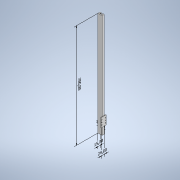
# Autodesk Inventor part: Guia
Saved by Autodesk Inventor 2021 (Build 250183000, 183)
## iProperties
Created: 2021-08-09
Part Number: Guia
Material: Generic
Document SubType Name: Modeling
Designer: guilh
Density: 1 g/cm^3
Appearance: Default
Author: guilh
Autodesk Inventor part; units mm, degrees
ref_plane "YZ Plane" through (0, 0, 0) normal (1, 0, 0) x (0, 1, 0)
ref_plane "XZ Plane" through (0, 0, 0) normal (0, 1, 0) x (-1, 0, 0)
ref_plane "XY Plane" through (0, 0, 0) normal (0, 0, 1) x (1, 0, 0)
sketch "Sketch1" plane through (0, 0, 0) normal (0, 1, 0) x (-1, 0, 0)
  line L0 (0, 0) -> (16, 0)
  line L1 (16, 0) -> (16, -5)
  line L2 (16, -5) -> (12, -5)
  line L3 (12, -5) -> (12, -10)
  line L4 (12, -10) -> (22, -10)
  line L5 (22, -10) -> (22, 5)
  line L6 (22, 5) -> (-4, 5)
  line L7 (0, 0) -> (0, -5)
  line L8 (0, -5) -> (4, -5)
  line L9 (4, -5) -> (4, -10)
  line L10 (4, -10) -> (-6, -10)
  line L11 (-6, -10) -> (-6, 5)
  line L12 (-6, 5) -> (-4, 5)
  dimension "d0" = 16
  dimension "d1" = 5
  dimension "d2" = 4
  dimension "d3" = 5
  dimension "d4" = 10
  dimension "d5" = 15
  dimension "d6" = 26
  dimension "d11" = 5
  dimension "d12" = 4
  dimension "d13" = 5
  dimension "d14" = 10
  dimension "d15" = 15
  constraints: 26 end point, 9 perpendicular, 2 vertical, 1 horizontal
  measures "d0" distance of L0.start L0.end
  measures "d1" distance of L0.end L1.end
  measures "d2" distance of L1.end L2.end
  measures "d3" distance of L2.end L3.end
  measures "d4" distance of L3.end L4.end
  measures "d5" distance of L4.end L5.end
  measures "d6" distance of L5.end L6.end
  measures "d11" distance of L0.start L7.end
  measures "d12" distance of L7.end L8.end
  measures "d13" distance of L8.end L9.end
  measures "d14" distance of L9.end L10.end
  measures "d15" distance of L10.end L11.end
extrude "Extrusion1" add sketch "Sketch1" along normal blind 500
sketch "Sketch2" plane through (6, 0, 5) normal (1, 0, 0) x (0, 0, -1)
  line L0 (0, 0) -> (0, 500) projected
  line L1 (0, 0) -> (0, 80)
  line L2 (0, 80) -> (15, 80)
  line L3 (15, 0) -> (15, 500) projected
  line L4 (15, 80) -> (35, 80)
  line L5 (35, 80) -> (35, 110)
  line L6 (35, 110) -> (-20, 110)
  line L7 (-20, 110) -> (-20, 50)
  line L8 (-20, 50) -> (35, 50)
  line L9 (35, 50) -> (35, 80)
  line L10 (-20, 110) -> (-10, 110)
  line L11 (-10, 110) -> (-10, 90)
  line L12 (-10, 90) -> (-10, 70)
  line L13 (-10, 70) -> (25, 70)
  line L14 (25, 70) -> (25, 90)
  line L15 (-10, 95) -> (-15.9639, 95)
  line L16 (-10, 65) -> (-17.5959, 65)
  circle A0 centre (25, 95) radius 5
  circle A1 centre (-10, 95) radius 5
  circle A2 centre (25, 65) radius 5
  circle A3 centre (-10, 65) radius 5
  point P0 (5, 0)
  dimension "d18" = 80
  dimension "d19" = 15
  dimension "d20" = 20
  dimension "d21" = 30
  dimension "d22" = 55
  dimension "d23" = 60
  dimension "d24" = 10
  dimension "d25" = 20
  dimension "d26" = 20
  dimension "d27" = 35
  dimension "d28" = 20
  dimension "d33" = 10
  dimension "d34" = 10
  dimension "d35" = 10
  dimension "d36" = 10
  constraints: 30 end point, 8 perpendicular, 7 point on line, 4 centre point, 1 horizontal
  measures "d18" distance of L0.start L1.end
  measures "d19" distance of L1.end L2.end
  measures "d20" distance of L2.end L4.end
  measures "d21" distance of L4.end L5.end
  measures "d22" distance of L5.end L6.end
  measures "d23" distance of L6.end L7.end
  measures "d24" distance of L6.end L10.end
  measures "d25" distance of L10.end L11.end
  measures "d26" distance of L11.end L12.end
  measures "d27" distance of L12.end L13.end
  measures "d28" distance of L13.end L14.end
  measures "d33" diameter of A0
  measures "d34" diameter of A1
  measures "d35" diameter of A2
  measures "d36" diameter of A3
extrude "Extrusion2" add sketch "Sketch2" along normal blind 3 contours L8 L7 L6 L11 A1 L12 L13 L0 | L0 L13 L3 L8 | L13 L12 A1 L11 L6 L0 | L0 L2 L3 L13 | L3 L13 L14 L4 L9 L8 | L0 L6 L3 L2 | L3 L4 L14 L13 | L3 L6 L5 L4
sketch "Sketch3" plane through (6, 0, 5) normal (-1, 0, 0) x (0, 0, 1)
  line L0 (20, 50) -> (-35, 50) projected
  line L1 (-35, 50) -> (-35, 110) projected
  line L2 (-35, 50) -> (-35, 110)
  line L3 (-35, 110) -> (20, 110) projected
  line L4 (-35, 110) -> (20, 110)
  line L5 (20, 110) -> (20, 50) projected
  line L6 (20, 110) -> (20, 50)
  line L7 (20, 50) -> (-35, 50)
  point P0 (-5, 0)
  constraints: 8 end point, 2 perpendicular, 1 collinear, 1 vertical
extrude "Extrusion3" add sketch "Sketch3" against normal blind 3
sketch "Sketch4" plane through (6, 0, 5) normal (-1, 0, 0) x (0, 0, 1)
  line L0 (0, 50) -> (0, 110) projected
  line L1 (0, 50) -> (9, 50)
  line L2 (20, 50) -> (-35, 50) projected
  line L3 (9, 50) -> (9, 110)
  line L4 (-35, 110) -> (20, 110) projected
  line L5 (9, 110) -> (23.2747, 110)
  line L6 (-35, 110) -> (-15, 110) projected
  line L7 (23.2747, 110) -> (23.2747, 50)
  line L8 (23.2747, 50) -> (9, 50)
  line L9 (-15, 50) -> (-35, 50) projected
  line L10 (-15, 50) -> (-24, 50)
  line L11 (-24, 50) -> (-24, 110)
  line L12 (-24, 110) -> (-51.0156, 108.7427)
  line L13 (-51.0156, 108.7427) -> (-51.1782, 112.2347)
  line L14 (-51.1782, 112.2347) -> (-24, 110)
  line L15 (-51.0156, 108.7427) -> (-55.6093, 34.9275)
  line L16 (-55.6093, 34.9275) -> (-24, 50)
  point P0 (-5, 0)
  dimension "d41" = 9
  dimension "d42" = 9
  constraints: 24 end point, 5 point on line, 4 perpendicular, 2 collinear
  measures "d41" distance of L0.start L1.end
  measures "d42" distance of L9.start L10.end
extrude "Extrusion4" cut sketch "Sketch4" against normal blind 3 contours L3 L4 L5 L7 L8 L2 | L16 L15 L12 L11 | L12 L13 L14
sketch "Sketch5" plane through (6, 0, 5) normal (-1, 0, 0) x (0, 0, 1)
  line L0 (-15, 50) -> (-24, 50) projected
  line L1 (-24, 50) -> (-19.5, 50)
  circle A0 centre (-19.5, 95) radius 2.5
  circle A1 centre (-19.5, 80) radius 2.5
  circle A2 centre (-19.5, 65) radius 2.5
  line L2 (9, 50) -> (0, 50) projected
  line L3 (9, 50) -> (4.5, 50)
  circle A3 centre (4.5, 95) radius 2.5
  circle A4 centre (4.5, 80) radius 2.5
  circle A5 centre (4.5, 65) radius 2.5
  point P0 (-5, 0)
  dimension "d48" = 5
  dimension "d49" = 5
  dimension "d50" = 5
  dimension "d51" = 4.5
  dimension "d52" = 5
  dimension "d53" = 5
  dimension "d54" = 5
  constraints: 6 centre point, 4 end point, 2 midpoint
  measures "d48" diameter of A0
  measures "d49" diameter of A1
  measures "d50" diameter of A2
  measures "d51" distance of L2.start L3.end
  measures "d52" diameter of A3
  measures "d53" diameter of A4
  measures "d54" diameter of A5
extrude "Extrusion5" cut sketch "Sketch5" against normal blind 3
thicken "Thicken1" operation add thickness 200 both sides no extend neighbours yes toward (0, 1, 0) faces at (-5.3333, 500, 3.3333)
body "Solid1"
